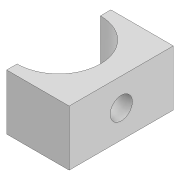
# Autodesk Inventor part: Tube_adaptor
Saved by Autodesk Inventor 2022 (Build 260153000, 153)
## iProperties
Created: 2022-05-02
Part Number: Tube_adaptor
Material: Generic
Document SubType Name: Modeling
Designer: dell
Density: 1 g/cm^3
Appearance: Default
Author: dell
Autodesk Inventor part; units mm, degrees
ref_plane "YZ Plane" through (0, 0, 0) normal (1, 0, 0) x (0, 1, 0)
ref_plane "XZ Plane" through (0, 0, 0) normal (0, 1, 0) x (-1, 0, 0)
ref_plane "XY Plane" through (0, 0, 0) normal (0, 0, 1) x (1, 0, 0)
sketch "Sketch1" plane through (0, 0, 0) normal (0, 1, 0) x (-1, 0, 0)
  line L0 (0, 0) -> (9, 0)
  line L1 (9, 0) -> (9, -15)
  line L2 (9, -15) -> (0, -15)
  line L3 (0, -15) -> (0, 0)
  circle A0 centre (9, -7.5) radius 6
  point P0 (9, -13.5)
  point P1 (9, -1.5)
  dimension "d1" = 9
  dimension "d7" = 15
  dimension "d8" = 15
  dimension "d9" = 12
  constraints: 8 end point, 1 centre point, 1 horizontal, 1 midpoint, 1 parallel, 1 perpendicular
  measures "d1" distance between parallel lines of L1 L3
  measures "d7" distance of L2.end L0.start
  measures "d8" distance of L0.end L1.end
  measures "d9" diameter of A0
extrude "Extrusion1" add sketch "Sketch1" along normal blind 8 contours L0 L1 A0 L2 L3
sketch "Sketch2" plane through (0, 0, 0) normal (1, 0, 0) x (0, 0, -1)
  circle A0 centre (7.5, 4) radius 1.6
  line L0 (0, 0) -> (15, 0) projected
  line L1 (0, 0) -> (0, 8) projected
  dimension "d4" = 3.2
  dimension "d5" = 4
  dimension "d6" = 7.5
  constraints: 1 centre point
  measures "d4" diameter of A0
  measures "d5" distance from line of L0 A0.centre
  measures "d6" distance from line of L1 A0.centre
extrude "Extrusion2" cut sketch "Sketch2" against normal blind 6
body "Solid1"
